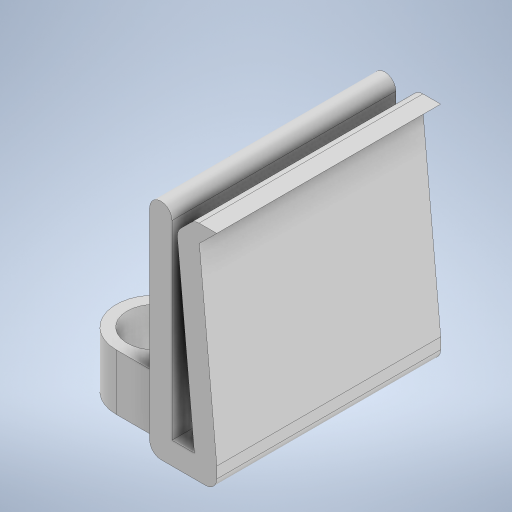
# Autodesk Inventor part: theWritersHolster
Saved by Autodesk Inventor 2024 (Build 280153000, 153)
## iProperties
Created: 2023-09-19
Part Number: theWritersHolster
Material: Generic
Document SubType Name: Modeling
Designer: afraz
Density: 1 g/cm^3
Appearance: Default
Author: afraz
Autodesk Inventor part; units mm, degrees
ref_plane "YZ Plane" through (0, 0, 0) normal (1, 0, 0) x (0, 1, 0)
ref_plane "XZ Plane" through (0, 0, 0) normal (0, 1, 0) x (-1, 0, 0)
ref_plane "XY Plane" through (0, 0, 0) normal (0, 0, 1) x (1, 0, 0)
sketch "Sketch1" plane through (0, 0, 0) normal (0, 1, 0) x (-1, 0, 0)
  line L0 (0, 0) -> (-12, 0)
  line L1 (-12, 0) -> (-12, -40)
  line L2 (-12, -40) -> (0, -40)
  line L3 (0, -40) -> (0, 0)
  point P0 (-6, 0)
  dimension "d0" = 40
  dimension "d1" = 12
  constraints: 8 end point, 2 parallel, 1 horizontal, 1 midpoint, 1 perpendicular
  measures "d0" distance from line of L2 point (-6, 0)
  measures "d1" distance between parallel lines of L3 L1
extrude "Extrusion1" add sketch "Sketch1" along normal blind 40
sketch "Sketch2" plane through (12, 0, -40) normal (0, 0, -1) x (-1, 0, 0)
  line L0 (0, 40) -> (12, 40) projected
  line L1 (8, 40) -> (8, 4)
  line L2 (8, 4) -> (4, 4)
  line L3 (4, 4) -> (7.129, 36.8805)
  line L4 (7.129, 36.8805) -> (4, 40)
  line L5 (4, 40) -> (8, 40)
  line L6 (12, 0) -> (12, 40) projected
  line L7 (0, 0) -> (0, 40) projected
  line L8 (0, 0) -> (12, 0) projected
  line L9 (0, 4) -> (3.129, 36.8805)
  line L10 (3.129, 36.8805) -> (0, 40)
  point P0 (6, 0)
  point P1 (6, 4)
  dimension "d4" = 4
  dimension "d5" = 4
  dimension "d6" = 4
  dimension "d7" = 4
  dimension "d8" = 4
  dimension "d9" = 4
  dimension "d10" = 3.982
  dimension "d11" = 2.8241
  constraints: 14 end point, 2 midpoint, 2 parallel, 2 point on line, 1 perpendicular, 1 vertical
  measures "d4" distance between parallel lines of L1 L6
  measures "d5" distance from line of L7 L2.end
  measures "d6" distance of point (6, 0) point (6, 4)
  measures "d7" distance of L9.start L2.end
  measures "d8" distance of L9.end L3.end
  measures "d9" distance of L0.start L4.end
  measures "d10" distance between parallel lines of L9 L3
  measures "d11" distance between parallel lines of L10 L4
extrude "Extrusion2" cut sketch "Sketch2" against normal blind 40 contours L10 L9 L7 | L0 L1 L2 L3 L4
fillet "Fillet1" radius 2 6 edges at (12, 0, -20) (0, 0, -20) (0, 40, -20) (4, 40, -20) (8, 40, -20) (4.871, 36.8805, -20)
sketch "Sketch3" plane through (0, 2, -40) normal (-1, 0, 0) x (0, 0, 1)
  line L0 (40, 0) -> (0, 0) projected
  line L1 (39, 0) -> (1, 0)
  line L2 (1, 0) -> (1, 10)
  line L3 (1, 10) -> (39, 10)
  line L4 (39, 10) -> (39, 0)
  line L5 (0, 0) -> (0, 36) projected
  point P0 (40, -2)
  point P1 (1, 0)
  dimension "d15" = 38
  dimension "d16" = 1
  dimension "d17" = 10
  constraints: 8 end point, 2 parallel, 1 horizontal, 1 perpendicular, 1 point on line
  measures "d15" distance between parallel lines of L2 L4
  measures "d16" distance between parallel lines of L5 L2
  measures "d17" distance between parallel lines of L3 L0
extrude "Extrusion3" add sketch "Sketch3" along normal blind 14
sketch "Sketch4" plane through (-14, 2, -1) normal (0, -1, 0) x (1, 0, 0)
  circle A0 centre (7, -7) radius 5
  circle A1 centre (7, -31) radius 5
  circle A2 centre (7, -19) radius 5
  line L0 (14, -38) -> (0, -38) projected
  line L1 (0, -38) -> (0, 0) projected
  point P0 (14, 1)
  point P1 (0, -19)
  dimension "d20" = 10
  dimension "d21" = 10
  dimension "d22" = 10
  dimension "d23" = 2
  dimension "d24" = 2
  dimension "d25" = 2
  dimension "d26" = 7
  dimension "d27" = 7
  dimension "d28" = 7
  constraints: 3 centre point, 1 midpoint
  measures "d20" diameter of A1
  measures "d21" diameter of A2
  measures "d22" diameter of A0
  measures "d23" distance edge to line of A1 L0
  measures "d26" distance from line of L1 A1.centre
  measures "d27" distance of point (0, -19) A2.centre
  measures "d28" distance from line of L1 A0.centre
extrude "Extrusion4" cut sketch "Sketch4" against normal blind 14
fillet "Fillet2" radius 7 1 edges at (-14, 7, -39)
fillet "Fillet3" radius 7 1 edges at (-14, 7, -1)
sketch "Sketch5" plane through (0, 2, -39) normal (0, -1, 0) x (1, 0, 0)
  circle A0 centre (-7, 19) radius 5 projected
  arc A1 (-14, 7) -> (-7, 0) centre (-7, 7) ccw projected
  arc A2 (-10.6056, 13) -> (-14, 7) centre (-7, 7) ccw
  line L0 (-14, 7) -> (-14, 31) projected
  circle A3 centre (-7, 7) radius 5 projected
  arc A4 (-14, 19) -> (-10.6056, 13) centre (-7, 19) ccw
  circle A5 centre (-7, 31) radius 5 projected
  arc A6 (-10.6056, 25) -> (-14, 19) centre (-7, 19) ccw
  arc A7 (-7, 38) -> (-14, 31) centre (-7, 31) ccw projected
  arc A8 (-14, 31) -> (-10.6056, 25) centre (-7, 31) ccw
  line L1 (-14, 31) -> (-14, 7)
  point P0 (0, 39)
  dimension "d33" = 7
  dimension "d34" = 7
  constraints: 8 point on circle, 4 centre point, 3 tangent, 2 end point, 1 collinear, 1 midpoint
  measures "d33" radius of A2
  measures "d34" radius of A4
extrude "Extrusion5" cut sketch "Sketch5" against normal blind 14 contours L0 A8 A6 | A2 L0 A4
body "Solid1"
